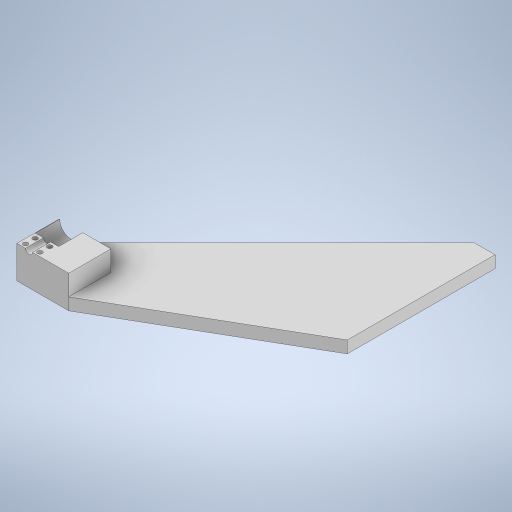
# Autodesk Inventor part: Z_babka
Saved by Autodesk Inventor 2024 (Build 280153000, 153)
## iProperties
Created: 2023-09-10
Part Number: Z_babka
Material: Generic
Document SubType Name: Modeling
Designer: KirikDK
Density: 1 g/cm^3
Appearance: Default
Author: KirikDK
Autodesk Inventor part; units mm, degrees
ref_plane "YZ Plane" through (0, 0, 0) normal (1, 0, 0) x (0, 1, 0)
ref_plane "XZ Plane" through (0, 0, 0) normal (0, 1, 0) x (-1, 0, 0)
ref_plane "XY Plane" through (0, 0, 0) normal (0, 0, 1) x (1, 0, 0)
sketch "Sketch1" plane through (0, 0, 0) normal (0, 1, 0) x (-1, 0, 0)
  line L0 (111.9461, 87.1683) -> (-118.0539, 87.1683)
  line L1 (-118.0539, 87.1683) -> (-118.0539, -87.8317)
  line L2 (-118.0539, -87.8317) -> (111.9461, -87.8317)
  line L3 (111.9461, -87.8317) -> (111.9461, 87.1683)
  line L4 (111.9461, 52.1683) -> (-28.0539, -87.8317)
  point P0 (0, 0)
  dimension "d0" = 175
  dimension "d1" = 230
  dimension "d2" = 45
  dimension "d3" = 35
  constraints: 10 end point, 2 parallel, 2 point on line, 1 horizontal, 1 perpendicular
  measures "d0" distance of L0.end L1.end
  measures "d1" distance of L0.start L0.end
  measures "d2" angle of L2 L4
  measures "d3" distance of L0.start L4.start
extrude "Extrusion1" add sketch "Sketch1" along normal blind 10 contours L3 L4 L2 L1 L0
sketch "Sketch2" plane through (0, 10, 0) normal (0, 1, 0) x (1, 0, 0)
  line L0 (-111.9461, -52.1683) -> (-111.9461, -87.1683) projected
  line L1 (-111.9461, -87.1683) -> (-69, -87.1683)
  line L2 (-69, -87.1683) -> (-69, -52.1683)
  line L3 (-69, -52.1683) -> (-111.9461, -52.1683)
  line L4 (-111.9461, -52.1683) -> (-111.9461, -87.1683)
  point P0 (0, 0)
  constraints: 8 end point, 2 parallel, 1 horizontal, 1 perpendicular
extrude "Extrusion2" add sketch "Sketch2" along normal blind 17
sketch "Sketch3" plane through (-111.9461, 0, 87.1683) normal (0, 0, 1) x (1, 0, 0)
  line L0 (0, 27) -> (42.9461, 27) projected
  circle A0 centre (10, 27) radius 2.9
  point P0 (111.9461, 0)
  point P1 (12.9, 27)
  point P2 (7.1, 27)
  dimension "d12" = 5.8
  constraints: 1 centre point, 1 point on line
  measures "d12" diameter of A0
extrude "Extrusion3" cut sketch "Sketch3" against normal blind 40 contours L0 A0 picked at (10.9386, 26.7687)
sketch "Sketch4" plane through (-69, 10, 52.1683) normal (0, 0, -1) x (-1, 0, 0)
  arc A0 (30.0461, 17) -> (35.8461, 17) centre (32.9461, 17) ccw projected
  circle A1 centre (32.9461, 17) radius 9.6071
  point P0 (-69, -10)
  constraints: 1 centre point, 1 coincident
extrude "Extrusion4" cut sketch "Sketch4" against normal blind 20
sketch "Sketch5" plane through (0, 27, 0) normal (0, 1, 0) x (1, 0, 0)
  circle A0 centre (-108, -84) radius 2
  circle A1 centre (-108, -76) radius 2
  circle A2 centre (-96, -76) radius 2
  circle A3 centre (-96, -84) radius 2
  point P0 (0, 0)
  constraints: 4 centre point
extrude "Extrusion5" cut sketch "Sketch5" against normal blind 40
sketch "Sketch6" plane through (0, 10, 0) normal (0, 1, 0) x (1, 0, 0)
  line L0 (-111.9461, -87.1683) -> (118.0539, -87.1683) projected
  line L1 (118.0539, -87.1683) -> (118.0539, 87.8317) projected
  line L2 (-99.0461, -87.1683) -> (-69, -87.1683) projected
  line L3 (-69, -87.1683) -> (118.0539, 20.8273)
  point P0 (0, 0)
  dimension "d18" = 30
  constraints: 2 end point, 1 point on line
  measures "d18" angle of L0 L3
extrude "Extrusion6" cut sketch "Sketch6" against normal blind 40
sketch "Sketch7" plane through (0, 10, 0) normal (0, 1, 0) x (1, 0, 0)
  line L0 (28.0539, 87.8317) -> (-111.9461, -52.1683) projected
  line L1 (28.0539, 87.8317) -> (93.621, 153.3988)
  line L2 (93.621, 153.3988) -> (118.0539, 153.3988)
  line L3 (118.0539, 20.8273) -> (118.0539, 87.8317) projected
  line L4 (118.0539, 153.3988) -> (118.0539, 87.8317)
  line L5 (28.0539, 87.8317) -> (118.0539, 87.8317)
  point P0 (0, 0)
  constraints: 8 end point, 2 horizontal, 1 collinear
extrude "Extrusion7" add sketch "Sketch7" against normal blind 10
sketch "Sketch8" plane through (0, 10, 0) normal (0, 1, 0) x (1, 0, 0)
  line L0 (118.0539, 20.8273) -> (118.0539, 153.3988) projected
  line L1 (118.0539, 153.3988) -> (77.5539, 153.3988)
  line L2 (77.5539, 153.3988) -> (77.5539, -53)
  line L3 (77.5539, -53) -> (118.0539, -53)
  line L4 (118.0539, -53) -> (118.0539, 153.3988)
  line L5 (77.5539, 153.3988) -> (12, 153.3988)
  line L6 (12, 153.3988) -> (12, 120)
  line L7 (12, 120) -> (77.5539, 120)
  line L8 (77.5539, 120) -> (77.5539, 153.3988)
  point P0 (0, 0)
  dimension "d23" = 40.5
  constraints: 16 end point, 4 parallel, 2 horizontal, 2 perpendicular
  measures "d23" distance between parallel lines of L2 L0
extrude "Extrusion8" cut sketch "Sketch8" against normal blind 10
body "Solid1"
